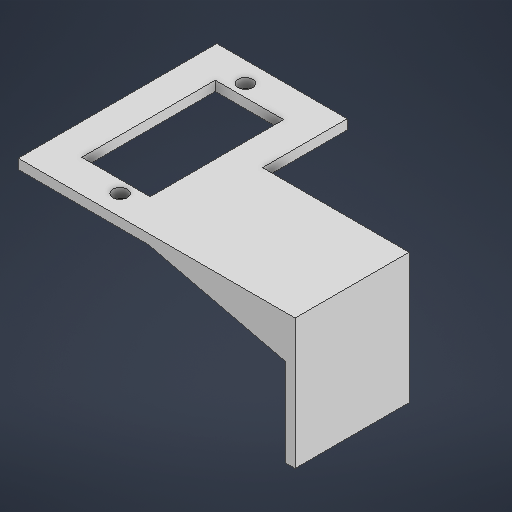
# Autodesk Inventor part: pan_base_holder_second
Saved by Autodesk Inventor 2026 (Build 300175000, 175)
## iProperties
Created: 2025-06-27
Part Number: pan_base_holder_second
Material: Generic
Document SubType Name: Modeling
Designer: user
Density: 1 g/cm^3
Appearance: Default
Author: user
Autodesk Inventor part; units mm, degrees
ref_plane "YZ Plane" through (0, 0, 0) normal (1, 0, 0) x (0, 1, 0)
ref_plane "XZ Plane" through (0, 0, 0) normal (0, 1, 0) x (-1, 0, 0)
ref_plane "XY Plane" through (0, 0, 0) normal (0, 0, 1) x (1, 0, 0)
sketch "Sketch1" plane through (0, 0, 0) normal (0, 0, 1) x (1, 0, 0)
  line L0 (-31, -31) -> (31, -31)
  line L1 (31, -31) -> (31, 31)
  line L2 (31, 31) -> (-31, 31)
  line L3 (-31, 31) -> (-31, -31)
  line L4 (-31, -31) -> (31, 31) construction
  line L5 (31, -31) -> (-31, 31) construction
  line L6 (-33, 33) -> (33, 33)
  line L7 (33, 33) -> (33, -33)
  line L8 (33, -33) -> (-33, -33)
  line L9 (-33, -33) -> (-33, 33)
  point P0 (0, 0)
  dimension "d0" = 62
  dimension "d1" = 62
  dimension "d2" = 2
  constraints: 20 end point, 4 parallel, 2 midpoint, 2 perpendicular, 1 horizontal, 3 other
  measures "d0" distance of L1.end L2.end
  measures "d1" distance of L0.end L1.end
  measures "d2" distance between parallel lines of L2 L6
extrude "Extrusion1" add sketch "Sketch1" along normal blind 2 contours L3 L2 L1 L0 | L6 L7 L8 L9
extrude "Extrusion2" add sketch "Sketch1" against normal blind 12
sketch "Sketch2" plane through (-33, 33, 2) normal (0, 1, 0) x (1, 0, 0)
  line L0 (13, 3) -> (53, 3)
  line L1 (53, 3) -> (53, 0)
  line L2 (53, 0) -> (13, 0)
  line L3 (13, 0) -> (13, 3)
  line L4 (0, 14) -> (0, 0) projected
  line L5 (0, 14) -> (66, 14) projected
  point P0 (33, 2)
  dimension "d7" = 40
  dimension "d8" = 3
  dimension "d9" = 13
  dimension "d10" = 11
  constraints: 8 end point, 2 parallel, 1 horizontal, 1 perpendicular
  measures "d7" distance of L1.end L2.end
  measures "d8" distance of L0.end L1.end
  measures "d9" distance between parallel lines of L4 L3
  measures "d10" distance between parallel lines of L5 L0
extrude "Extrusion3" add sketch "Sketch2" along normal blind 12
sketch "Sketch3" plane through (20, 33, -1) normal (0, 0, -1) x (-1, 0, 0)
  line L0 (40, 12) -> (0, 12) projected
  line L1 (40, 0) -> (40, 12) projected
  line L2 (0, 12) -> (40, 12)
  line L3 (40, 12) -> (40, 9)
  line L4 (40, 9) -> (0, 9)
  line L5 (0, 9) -> (0, 12)
  point P0 (20, -33)
  dimension "d13" = 3
  constraints: 8 end point, 2 parallel, 1 horizontal, 1 perpendicular, 1 point on line
  measures "d13" distance of L2.end L3.end
extrude "Extrusion4" add sketch "Sketch3" along normal blind 80
sketch "Sketch4" plane through (-20, 42, -1) normal (0, -1, 0) x (1, 0, 0)
  line L0 (30.5, -63) -> (9.5, -63)
  line L1 (9.5, -63) -> (9.5, -22)
  line L2 (9.5, -22) -> (30.5, -22)
  line L3 (30.5, -22) -> (30.5, -63)
  line L4 (40, 3) -> (40, -80) projected
  line L5 (0, 3) -> (40, 3) projected
  point P0 (20, 1)
  dimension "d16" = 21
  dimension "d17" = 41
  dimension "d18" = 9.5
  dimension "d19" = 25
  constraints: 8 end point, 2 parallel, 1 horizontal, 1 perpendicular
  measures "d16" distance of L0.start L0.end
  measures "d17" distance of L0.end L1.end
  measures "d18" distance between parallel lines of L4 L3
  measures "d19" distance between parallel lines of L2 L5
extrude "Extrusion5" cut sketch "Sketch4" against normal blind 80
sketch "Sketch5" plane through (-20, 42, -1) normal (0, -1, 0) x (1, 0, 0)
  line L0 (30.5, -63) -> (9.5, -63) projected
  line L1 (30.5, -63) -> (9.5, -63)
  line L2 (9.5, -63) -> (9.5, -70)
  line L3 (9.5, -70) -> (30.5, -70)
  line L4 (30.5, -70) -> (30.5, -63)
  circle A0 centre (15, -66.75) radius 2.25
  line L5 (30.5, -22) -> (30.5, -63) projected
  line L6 (30.5, -22) -> (9.5, -22)
  line L7 (9.5, -22) -> (9.5, -15)
  line L8 (9.5, -15) -> (30.5, -15)
  line L9 (30.5, -15) -> (30.5, -22)
  circle A1 centre (25, -18.25) radius 2.25
  point P0 (20, 1)
  point P1 (15.4717, -69.81)
  point P2 (14.5283, -69.81)
  point P3 (24.5283, -15.19)
  point P4 (25.4717, -15.19)
  dimension "d22" = 7
  dimension "d23" = 4.5
  dimension "d24" = 3.75
  dimension "d25" = 5.5
  dimension "d26" = 7
  dimension "d27" = 4.5
  dimension "d28" = 5.5
  dimension "d29" = 3.75
  constraints: 16 end point, 4 parallel, 2 centre point, 2 horizontal, 2 perpendicular
  measures "d22" distance of L2.end L1.end
  measures "d23" diameter of A0
  measures "d24" distance from line of A0.centre L0
  measures "d25" distance from line of L2 A0.centre
  measures "d26" distance of L6.end L7.end
  measures "d27" diameter of A1
  measures "d28" distance from line of L9 A1.centre
  measures "d29" distance from line of L6 A1.centre
extrude "Extrusion6" cut sketch "Sketch5" against normal blind 80 contours A0 | A1
sketch "Sketch6" plane through (-33, -33, 2) normal (0, -1, 0) x (1, 0, 0)
  line L0 (0, 0) -> (66, 0) projected
  line L1 (66, -14) -> (0, -14) projected
  line L2 (0, 0) -> (66, 0)
  line L3 (66, 0) -> (66, -14)
  line L4 (66, -14) -> (0, -14)
  line L5 (0, -14) -> (0, 0)
  point P0 (33, -2)
  constraints: 8 end point, 2 parallel, 1 horizontal, 1 perpendicular
extrude "Extrusion7" cut sketch "Sketch6" against normal up to surface (75 mm away)
sketch "Sketch7" plane through (-20, 42, -81) normal (0, -1, 0) x (1, 0, 0)
  line L0 (40, 83) -> (40, 0) projected
  line L1 (40, 0) -> (85, 0)
  line L2 (85, 0) -> (85, 83)
  line L3 (85, 83) -> (40, 83)
  line L4 (40, 83) -> (40, 0)
  line L5 (85, 33) -> (40, 33)
  point P0 (20, 81)
  point P1 (40, 33)
  dimension "d34" = 45
  dimension "d35" = 83
  dimension "d36" = 50
  constraints: 10 end point, 2 parallel, 2 perpendicular, 2 point on line, 1 horizontal
  measures "d34" distance of L3.end L2.end
  measures "d35" distance of L2.end L1.end
  measures "d36" distance between parallel lines of L3 L5
extrude "Extrusion8" add sketch "Sketch7" against normal up to surface (3 mm away) contours L3 L2 L5 L0
sketch "Sketch8" plane through (-20, 42, -81) normal (0, -1, 0) x (1, 0, 0)
  line L0 (0, 83) -> (85, 83)
  line L1 (85, 83) -> (85, 0)
  line L2 (85, 0) -> (0, 0)
  line L3 (0, 0) -> (0, 83)
  line L4 (85, 7) -> (0, 7)
  line L5 (85, 33) -> (85, 83) projected
  line L6 (-12.2623, 85.093) -> (0, 83)
  line L7 (0, 83) -> (-11.5686, 87.0435)
  line L8 (-11.5686, 87.0435) -> (85, 70.5603)
  line L9 (0, 83) -> (100, 83)
  line L10 (100, 83) -> (100, 68)
  line L11 (100, 68) -> (0, 68)
  line L12 (0, 68) -> (0, 83)
  point P0 (20, 81)
  point P1 (0, 73.8499)
  point P2 (27.25, 61.75)
  point P3 (27.25, 61.75)
  point P4 (25.55, 64.81)
  point P5 (0, 68)
  point P6 (85, 68)
  dimension "d40" = 83
  dimension "d41" = 7
  dimension "d43" = 15
  constraints: 24 end point, 5 parallel, 5 point on line, 3 perpendicular, 2 horizontal, 2 other
  measures "d40" distance of L0.end L1.end
  measures "d41" distance between parallel lines of L4 L2
  measures "d43" distance of L9.end L10.end
extrude "Extrusion9" cut sketch "Sketch8" against normal blind 10 contours L0 L8 L1 L11 L3 | L0 L1 L8 | L4 L1 L2 L3
sketch "Sketch9" plane through (20, 42, -48) normal (0, -1, 0) x (1, 0, 0)
  line L0 (45, 0) -> (45, 35) projected
  line L1 (0, 0) -> (45, 0) projected
  line L2 (45, 35) -> (42, 35)
  line L3 (42, 35) -> (42, 0)
  line L4 (42, 0) -> (45, 0)
  line L5 (45, 0) -> (45, 35)
  point P0 (-20, 48)
  dimension "d46" = 3
  constraints: 8 end point, 2 parallel, 1 horizontal, 1 perpendicular, 1 point on line
  measures "d46" distance of L4.end L3.end
extrude "Extrusion10" add sketch "Sketch9" along normal blind 100
sketch "Sketch10" plane through (65, 45, -13) normal (1, 0, 0) x (0, 0, -1)
  circle A0 centre (18, -56.25) radius 2.125
  circle A1 centre (18, -93) radius 2.125
  circle A2 centre (18, -74.625) radius 6.45
  line L0 (20.093, -55.8824) -> (22.589, -70.0925)
  line L1 (15.9065, -55.8857) -> (13.439, -70.0643)
  line L2 (20.0935, -93.3643) -> (22.561, -79.1857)
  line L3 (15.8877, -93.2317) -> (13.411, -79.1575)
  line L4 (18, -56.25) -> (18, -74.625)
  line L5 (18, -74.625) -> (18, -93)
  line L6 (35, 0) -> (35, -103) projected
  line L7 (35, -103) -> (0, -103) projected
  point P0 (-13, -45)
  dimension "d49" = 4.25
  dimension "d50" = 4.25
  dimension "d51" = 12.9
  dimension "d52" = 9.15
  dimension "d53" = 9.15
  dimension "d54" = 41
  dimension "d57" = 17
  dimension "d58" = 10
  constraints: 12 end point, 8 point on circle, 3 centre point, 3 tangent, 2 vertical, 1 collinear
  measures "d49" diameter of A0
  measures "d50" diameter of A1
  measures "d51" diameter of A2
  measures "d52" distance of L1.end L0.end
  measures "d53" distance of L3.end L2.end
  measures "d57" distance from line of L6 L4.end
  measures "d58" distance from line of L7 L5.end
extrude "Extrusion11" cut sketch "Sketch10" against normal blind 2.5
sketch "Sketch11" plane through (65, 45, -13) normal (1, 0, 0) x (0, 0, -1)
  line L0 (35, -3) -> (35, -103) projected
  line L1 (0, 0) -> (0, -103) projected
  line L2 (35, -103) -> (0, -103)
  line L3 (0, -103) -> (0, 0)
  line L4 (0, 0) -> (35, 0)
  line L5 (35, 0) -> (35, -103)
  line L6 (35, -40) -> (0, -40)
  point P0 (-13, -45)
  dimension "d59" = 40
  constraints: 10 end point, 2 parallel, 2 perpendicular, 2 point on line, 1 horizontal
  measures "d59" distance between parallel lines of L4 L6
extrude "Extrusion12" cut sketch "Sketch11" against normal blind 10 contours L0 L2 L1 L6
sketch "Sketch12" plane through (65, 45, -48) normal (0, 0, -1) x (-1, 0, 0)
  line L0 (45, -3) -> (3, -3) projected
  line L1 (3, -3) -> (45, -3)
  line L2 (45, -3) -> (45, -13)
  line L3 (45, -13) -> (3, -13)
  line L4 (3, -13) -> (3, -3)
  line L5 (3, -13) -> (45, -3)
  point P0 (65, -45)
  dimension "d62" = 42
  dimension "d63" = 10
  constraints: 10 end point, 2 parallel, 1 horizontal, 1 perpendicular
  measures "d62" distance of L2.end L3.end
  measures "d63" distance of L1.end L2.end
extrude "Extrusion13" add sketch "Sketch12" against normal blind 2 contours L5 L4 L0
ref_plane "Work Plane1" through (65, 45, -30.5) normal (0, 0, -1) x (-1, 0, 0)
mirror "Mirror1" about plane through (65, 45, -30.5) normal (0, 0, -1) of "Extrusion13"
body "Solid1"
